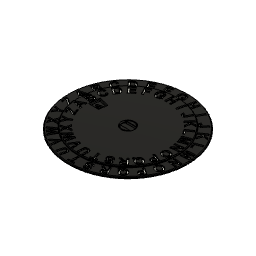
Decoder 2.0 v3 (Autodesk Fusion 360 design; units mm, degrees)
Autodesk Fusion 360 part; units mm, degrees
sketch "Sketch1" plane through (0, 0, 0) normal (0, 0, 1) x (1, 0, 0) in component "Decoder Base"
  line L0 (0, 0) -> (-75, 0)
  arc A0 (-72.8206, 17.9487) -> (-75, 0) centre (0, 0) ccw
  line L1 (0, 0) -> (-72.8206, 17.9487) construction
  line L2 (0, 0) -> (-75, 0) construction
  line L3 (-75, 0) -> (-62.5, 0)
  line L4 (-62.5, 0) -> (-50, 0)
  line L5 (-62.5, 0) -> (-61.5, 0)
  line L6 (-50, 0) -> (-37.5, 0)
  arc A1 (-60.6839, 14.9572) -> (-62.5, 0) centre (0, 0) ccw
  line L7 (0, 0) -> (-60.6839, 14.9572) construction
  line L8 (0, 0) -> (-62.5, 0) construction
  arc A2 (-48.5471, 11.9658) -> (-50, 0) centre (0, 0) ccw
  line L9 (0, 0) -> (-48.5471, 11.9658) construction
  line L10 (0, 0) -> (-50, 0) construction
  arc A3 (-36.4103, 8.9743) -> (-37.5, 0) centre (0, 0) ccw
  line L11 (0, 0) -> (-36.4103, 8.9743) construction
  line L12 (0, 0) -> (-37.5, 0) construction
  arc A4 (-59.7129, 14.7179) -> (-61.5, 0) centre (0, 0) ccw
  line L13 (0, 0) -> (-59.7129, 14.7179) construction
  line L14 (0, 0) -> (-61.5, 0) construction
  arc A5 (-61.5, 0) -> (-59.7129, -14.7179) centre (0, 0) ccw
  arc A6 (-50, 0) -> (-48.5471, -11.9658) centre (0, 0) ccw
  arc A7 (-37.5, 0) -> (-36.4103, -8.9743) centre (0, 0) ccw
  arc A8 (-62.5, 0) -> (-60.6839, -14.9572) centre (0, 0) ccw
  line L15 (-72.8206, -17.9487) -> (-60.6839, -14.9572)
  line L16 (-60.6839, -14.9572) -> (-59.7129, -14.7179)
  line L17 (-48.5471, -11.9658) -> (-36.4103, -8.9743)
  line L18 (-60.6839, -14.9572) -> (-48.5471, -11.9658)
  arc A9 (-75, 0) -> (-72.8206, -17.9487) centre (0, 0) ccw
  arc A10 (-59.7129, -14.7179) -> (-54.4555, -28.5805) centre (0, 0) ccw
  arc A11 (-48.5471, -11.9658) -> (-44.2728, -23.2362) centre (0, 0) ccw
  arc A12 (-36.4103, -8.9743) -> (-33.2046, -17.4271) centre (0, 0) ccw
  arc A13 (-60.6839, -14.9572) -> (-55.341, -29.0452) centre (0, 0) ccw
  line L19 (-66.4092, -34.8542) -> (-55.341, -29.0452)
  line L20 (-55.341, -29.0452) -> (-54.4555, -28.5805)
  line L21 (-44.2728, -23.2362) -> (-33.2046, -17.4271)
  line L22 (-55.341, -29.0452) -> (-44.2728, -23.2362)
  arc A14 (-72.8206, -17.9487) -> (-66.4092, -34.8542) centre (0, 0) ccw
  arc A15 (-54.4555, -28.5805) -> (-46.0334, -40.782) centre (0, 0) ccw
  arc A16 (-44.2728, -23.2362) -> (-37.4255, -33.1561) centre (0, 0) ccw
  arc A17 (-33.2046, -17.4271) -> (-28.0692, -24.8671) centre (0, 0) ccw
  arc A18 (-55.341, -29.0452) -> (-46.7819, -41.4452) centre (0, 0) ccw
  line L23 (-56.1383, -49.7342) -> (-46.7819, -41.4452)
  line L24 (-46.7819, -41.4452) -> (-46.0334, -40.782)
  line L25 (-37.4255, -33.1561) -> (-28.0692, -24.8671)
  line L26 (-46.7819, -41.4452) -> (-37.4255, -33.1561)
  arc A19 (-66.4092, -34.8542) -> (-56.1383, -49.7342) centre (0, 0) ccw
  arc A20 (-46.0334, -40.782) -> (-34.936, -50.6135) centre (0, 0) ccw
  arc A21 (-37.4255, -33.1561) -> (-28.4032, -41.1492) centre (0, 0) ccw
  arc A22 (-28.0692, -24.8671) -> (-21.3024, -30.8619) centre (0, 0) ccw
  arc A23 (-46.7819, -41.4452) -> (-35.504, -51.4365) centre (0, 0) ccw
  line L27 (-42.6049, -61.7238) -> (-35.504, -51.4365)
  line L28 (-35.504, -51.4365) -> (-34.936, -50.6135)
  line L29 (-28.4032, -41.1492) -> (-21.3024, -30.8619)
  line L30 (-35.504, -51.4365) -> (-28.4032, -41.1492)
  arc A24 (-56.1383, -49.7342) -> (-42.6049, -61.7238) centre (0, 0) ccw
  arc A25 (-34.936, -50.6135) -> (-21.8082, -57.5035) centre (0, 0) ccw
  arc A26 (-28.4032, -41.1492) -> (-17.7302, -46.7508) centre (0, 0) ccw
  arc A27 (-21.3024, -30.8619) -> (-13.2977, -35.0631) centre (0, 0) ccw
  arc A28 (-35.504, -51.4365) -> (-22.1628, -58.4385) centre (0, 0) ccw
  line L31 (-26.5954, -70.1262) -> (-22.1628, -58.4385)
  line L32 (-22.1628, -58.4385) -> (-21.8082, -57.5035)
  line L33 (-17.7302, -46.7508) -> (-13.2977, -35.0631)
  line L34 (-22.1628, -58.4385) -> (-17.7302, -46.7508)
  arc A29 (-42.6049, -61.7238) -> (-26.5954, -70.1262) centre (0, 0) ccw
  arc A30 (-21.8082, -57.5035) -> (-7.413, -61.0516) centre (0, 0) ccw
  arc A31 (-17.7302, -46.7508) -> (-6.0268, -49.6354) centre (0, 0) ccw
  arc A32 (-13.2977, -35.0631) -> (-4.5201, -37.2266) centre (0, 0) ccw
  arc A33 (-22.1628, -58.4385) -> (-7.5335, -62.0443) centre (0, 0) ccw
  line L35 (-9.0403, -74.4532) -> (-7.5335, -62.0443)
  line L36 (-7.5335, -62.0443) -> (-7.413, -61.0516)
  line L37 (-6.0268, -49.6354) -> (-4.5201, -37.2266)
  line L38 (-7.5335, -62.0443) -> (-6.0268, -49.6354)
  arc A34 (-26.5954, -70.1262) -> (-9.0403, -74.4532) centre (0, 0) ccw
  arc A35 (-7.413, -61.0516) -> (7.413, -61.0516) centre (0, 0) ccw
  arc A36 (-6.0268, -49.6354) -> (6.0268, -49.6354) centre (0, 0) ccw
  arc A37 (-4.5201, -37.2266) -> (4.5201, -37.2266) centre (0, 0) ccw
  arc A38 (-7.5335, -62.0443) -> (7.5335, -62.0443) centre (0, 0) ccw
  line L39 (9.0403, -74.4532) -> (7.5335, -62.0443)
  line L40 (7.5335, -62.0443) -> (7.413, -61.0516)
  line L41 (6.0268, -49.6354) -> (4.5201, -37.2266)
  line L42 (7.5335, -62.0443) -> (6.0268, -49.6354)
  arc A39 (-9.0403, -74.4532) -> (9.0403, -74.4532) centre (0, 0) ccw
  arc A40 (7.413, -61.0516) -> (21.8082, -57.5035) centre (0, 0) ccw
  arc A41 (6.0268, -49.6354) -> (17.7302, -46.7508) centre (0, 0) ccw
  arc A42 (4.5201, -37.2266) -> (13.2977, -35.0631) centre (0, 0) ccw
  arc A43 (7.5335, -62.0443) -> (22.1628, -58.4385) centre (0, 0) ccw
  line L43 (26.5954, -70.1262) -> (22.1628, -58.4385)
  line L44 (22.1628, -58.4385) -> (21.8082, -57.5035)
  line L45 (17.7302, -46.7508) -> (13.2977, -35.0631)
  line L46 (22.1628, -58.4385) -> (17.7302, -46.7508)
  arc A44 (9.0403, -74.4532) -> (26.5954, -70.1262) centre (0, 0) ccw
  arc A45 (21.8082, -57.5035) -> (34.936, -50.6135) centre (0, 0) ccw
  arc A46 (17.7302, -46.7508) -> (28.4032, -41.1492) centre (0, 0) ccw
  arc A47 (13.2977, -35.0631) -> (21.3024, -30.8619) centre (0, 0) ccw
  arc A48 (22.1628, -58.4385) -> (35.504, -51.4365) centre (0, 0) ccw
  line L47 (42.6049, -61.7238) -> (35.504, -51.4365)
  line L48 (35.504, -51.4365) -> (34.936, -50.6135)
  line L49 (28.4032, -41.1492) -> (21.3024, -30.8619)
  line L50 (35.504, -51.4365) -> (28.4032, -41.1492)
  arc A49 (26.5954, -70.1262) -> (42.6049, -61.7238) centre (0, 0) ccw
  arc A50 (34.936, -50.6135) -> (46.0334, -40.782) centre (0, 0) ccw
  arc A51 (28.4032, -41.1492) -> (37.4255, -33.1561) centre (0, 0) ccw
  arc A52 (21.3024, -30.8619) -> (28.0692, -24.8671) centre (0, 0) ccw
  arc A53 (35.504, -51.4365) -> (46.7819, -41.4452) centre (0, 0) ccw
  line L51 (56.1383, -49.7342) -> (46.7819, -41.4452)
  line L52 (46.7819, -41.4452) -> (46.0334, -40.782)
  line L53 (37.4255, -33.1561) -> (28.0692, -24.8671)
  line L54 (46.7819, -41.4452) -> (37.4255, -33.1561)
  arc A54 (42.6049, -61.7238) -> (56.1383, -49.7342) centre (0, 0) ccw
  arc A55 (46.0334, -40.782) -> (54.4555, -28.5805) centre (0, 0) ccw
  arc A56 (37.4255, -33.1561) -> (44.2728, -23.2362) centre (0, 0) ccw
  arc A57 (28.0692, -24.8671) -> (33.2046, -17.4271) centre (0, 0) ccw
  arc A58 (46.7819, -41.4452) -> (55.341, -29.0452) centre (0, 0) ccw
  line L55 (66.4092, -34.8542) -> (55.341, -29.0452)
  line L56 (55.341, -29.0452) -> (54.4555, -28.5805)
  line L57 (44.2728, -23.2362) -> (33.2046, -17.4271)
  line L58 (55.341, -29.0452) -> (44.2728, -23.2362)
  arc A59 (56.1383, -49.7342) -> (66.4092, -34.8542) centre (0, 0) ccw
  arc A60 (54.4555, -28.5805) -> (59.7129, -14.7179) centre (0, 0) ccw
  arc A61 (44.2728, -23.2362) -> (48.5471, -11.9658) centre (0, 0) ccw
  arc A62 (33.2046, -17.4271) -> (36.4103, -8.9743) centre (0, 0) ccw
  arc A63 (55.341, -29.0452) -> (60.6839, -14.9572) centre (0, 0) ccw
  line L59 (72.8206, -17.9487) -> (60.6839, -14.9572)
  line L60 (60.6839, -14.9572) -> (59.7129, -14.7179)
  line L61 (48.5471, -11.9658) -> (36.4103, -8.9743)
  line L62 (60.6839, -14.9572) -> (48.5471, -11.9658)
  arc A64 (66.4092, -34.8542) -> (72.8206, -17.9487) centre (0, 0) ccw
  arc A65 (59.7129, -14.7179) -> (61.5, 0) centre (0, 0) ccw
  arc A66 (48.5471, -11.9658) -> (50, 0) centre (0, 0) ccw
  arc A67 (36.4103, -8.9743) -> (37.5, 0) centre (0, 0) ccw
  arc A68 (60.6839, -14.9572) -> (62.5, 0) centre (0, 0) ccw
  line L63 (75, 0) -> (62.5, 0)
  line L64 (62.5, 0) -> (61.5, 0)
  line L65 (50, 0) -> (37.5, 0)
  line L66 (62.5, 0) -> (50, 0)
  arc A69 (72.8206, -17.9487) -> (75, 0) centre (0, 0) ccw
  arc A70 (61.5, 0) -> (59.7129, 14.7179) centre (0, 0) ccw
  arc A71 (50, 0) -> (48.5471, 11.9658) centre (0, 0) ccw
  arc A72 (37.5, 0) -> (36.4103, 8.9743) centre (0, 0) ccw
  arc A73 (62.5, 0) -> (60.6839, 14.9572) centre (0, 0) ccw
  line L67 (72.8206, 17.9487) -> (60.6839, 14.9572)
  line L68 (60.6839, 14.9572) -> (59.7129, 14.7179)
  line L69 (48.5471, 11.9658) -> (36.4103, 8.9743)
  line L70 (60.6839, 14.9572) -> (48.5471, 11.9658)
  arc A74 (75, 0) -> (72.8206, 17.9487) centre (0, 0) ccw
  arc A75 (59.7129, 14.7179) -> (54.4555, 28.5805) centre (0, 0) ccw
  arc A76 (48.5471, 11.9658) -> (44.2728, 23.2362) centre (0, 0) ccw
  arc A77 (36.4103, 8.9743) -> (33.2046, 17.4271) centre (0, 0) ccw
  arc A78 (60.6839, 14.9572) -> (55.341, 29.0452) centre (0, 0) ccw
  line L71 (66.4092, 34.8542) -> (55.341, 29.0452)
  line L72 (55.341, 29.0452) -> (54.4555, 28.5805)
  line L73 (44.2728, 23.2362) -> (33.2046, 17.4271)
  line L74 (55.341, 29.0452) -> (44.2728, 23.2362)
  arc A79 (72.8206, 17.9487) -> (66.4092, 34.8542) centre (0, 0) ccw
  arc A80 (54.4555, 28.5805) -> (46.0334, 40.782) centre (0, 0) ccw
  arc A81 (44.2728, 23.2362) -> (37.4255, 33.1561) centre (0, 0) ccw
  arc A82 (33.2046, 17.4271) -> (28.0692, 24.8671) centre (0, 0) ccw
  arc A83 (55.341, 29.0452) -> (46.7819, 41.4452) centre (0, 0) ccw
  line L75 (56.1383, 49.7342) -> (46.7819, 41.4452)
  line L76 (46.7819, 41.4452) -> (46.0334, 40.782)
  line L77 (37.4255, 33.1561) -> (28.0692, 24.8671)
  line L78 (46.7819, 41.4452) -> (37.4255, 33.1561)
  arc A84 (66.4092, 34.8542) -> (56.1383, 49.7342) centre (0, 0) ccw
  arc A85 (46.0334, 40.782) -> (34.936, 50.6135) centre (0, 0) ccw
  arc A86 (37.4255, 33.1561) -> (28.4032, 41.1492) centre (0, 0) ccw
  arc A87 (28.0692, 24.8671) -> (21.3024, 30.8619) centre (0, 0) ccw
  arc A88 (46.7819, 41.4452) -> (35.504, 51.4365) centre (0, 0) ccw
  line L79 (42.6049, 61.7238) -> (35.504, 51.4365)
  line L80 (35.504, 51.4365) -> (34.936, 50.6135)
  line L81 (28.4032, 41.1492) -> (21.3024, 30.8619)
  line L82 (35.504, 51.4365) -> (28.4032, 41.1492)
  arc A89 (56.1383, 49.7342) -> (42.6049, 61.7238) centre (0, 0) ccw
  arc A90 (34.936, 50.6135) -> (21.8082, 57.5035) centre (0, 0) ccw
  arc A91 (28.4032, 41.1492) -> (17.7302, 46.7508) centre (0, 0) ccw
  arc A92 (21.3024, 30.8619) -> (13.2977, 35.0631) centre (0, 0) ccw
  arc A93 (35.504, 51.4365) -> (22.1628, 58.4385) centre (0, 0) ccw
  line L83 (26.5954, 70.1262) -> (22.1628, 58.4385)
  line L84 (22.1628, 58.4385) -> (21.8082, 57.5035)
  line L85 (17.7302, 46.7508) -> (13.2977, 35.0631)
  line L86 (22.1628, 58.4385) -> (17.7302, 46.7508)
  arc A94 (42.6049, 61.7238) -> (26.5954, 70.1262) centre (0, 0) ccw
  arc A95 (21.8082, 57.5035) -> (7.413, 61.0516) centre (0, 0) ccw
  arc A96 (17.7302, 46.7508) -> (6.0268, 49.6354) centre (0, 0) ccw
  arc A97 (13.2977, 35.0631) -> (4.5201, 37.2266) centre (0, 0) ccw
  arc A98 (22.1628, 58.4385) -> (7.5335, 62.0443) centre (0, 0) ccw
  line L87 (9.0403, 74.4532) -> (7.5335, 62.0443)
  line L88 (7.5335, 62.0443) -> (7.413, 61.0516)
  line L89 (6.0268, 49.6354) -> (4.5201, 37.2266)
  line L90 (7.5335, 62.0443) -> (6.0268, 49.6354)
  arc A99 (26.5954, 70.1262) -> (9.0403, 74.4532) centre (0, 0) ccw
  arc A100 (7.413, 61.0516) -> (-7.413, 61.0516) centre (0, 0) ccw
  arc A101 (6.0268, 49.6354) -> (-6.0268, 49.6354) centre (0, 0) ccw
  arc A102 (4.5201, 37.2266) -> (-4.5201, 37.2266) centre (0, 0) ccw
  arc A103 (7.5335, 62.0443) -> (-7.5335, 62.0443) centre (0, 0) ccw
  line L91 (-9.0403, 74.4532) -> (-7.5335, 62.0443)
  line L92 (-7.5335, 62.0443) -> (-7.413, 61.0516)
  line L93 (-6.0268, 49.6354) -> (-4.5201, 37.2266)
  line L94 (-7.5335, 62.0443) -> (-6.0268, 49.6354)
  arc A104 (9.0403, 74.4532) -> (-9.0403, 74.4532) centre (0, 0) ccw
  arc A105 (-7.413, 61.0516) -> (-21.8082, 57.5035) centre (0, 0) ccw
  arc A106 (-6.0268, 49.6354) -> (-17.7302, 46.7508) centre (0, 0) ccw
  arc A107 (-4.5201, 37.2266) -> (-13.2977, 35.0631) centre (0, 0) ccw
  arc A108 (-7.5335, 62.0443) -> (-22.1628, 58.4385) centre (0, 0) ccw
  line L95 (-26.5954, 70.1262) -> (-22.1628, 58.4385)
  line L96 (-22.1628, 58.4385) -> (-21.8082, 57.5035)
  line L97 (-17.7302, 46.7508) -> (-13.2977, 35.0631)
  line L98 (-22.1628, 58.4385) -> (-17.7302, 46.7508)
  arc A109 (-9.0403, 74.4532) -> (-26.5954, 70.1262) centre (0, 0) ccw
  arc A110 (-21.8082, 57.5035) -> (-34.936, 50.6135) centre (0, 0) ccw
  arc A111 (-17.7302, 46.7508) -> (-28.4032, 41.1492) centre (0, 0) ccw
  arc A112 (-13.2977, 35.0631) -> (-21.3024, 30.8619) centre (0, 0) ccw
  arc A113 (-22.1628, 58.4385) -> (-35.504, 51.4365) centre (0, 0) ccw
  line L99 (-42.6049, 61.7238) -> (-35.504, 51.4365)
  line L100 (-35.504, 51.4365) -> (-34.936, 50.6135)
  line L101 (-28.4032, 41.1492) -> (-21.3024, 30.8619)
  line L102 (-35.504, 51.4365) -> (-28.4032, 41.1492)
  arc A114 (-26.5954, 70.1262) -> (-42.6049, 61.7238) centre (0, 0) ccw
  arc A115 (-34.936, 50.6135) -> (-46.0334, 40.782) centre (0, 0) ccw
  arc A116 (-28.4032, 41.1492) -> (-37.4255, 33.1561) centre (0, 0) ccw
  arc A117 (-21.3024, 30.8619) -> (-28.0692, 24.8671) centre (0, 0) ccw
  arc A118 (-35.504, 51.4365) -> (-46.7819, 41.4452) centre (0, 0) ccw
  line L103 (-56.1383, 49.7342) -> (-46.7819, 41.4452)
  line L104 (-46.7819, 41.4452) -> (-46.0334, 40.782)
  line L105 (-37.4255, 33.1561) -> (-28.0692, 24.8671)
  line L106 (-46.7819, 41.4452) -> (-37.4255, 33.1561)
  arc A119 (-42.6049, 61.7238) -> (-56.1383, 49.7342) centre (0, 0) ccw
  arc A120 (-46.0334, 40.782) -> (-54.4555, 28.5805) centre (0, 0) ccw
  arc A121 (-37.4255, 33.1561) -> (-44.2728, 23.2362) centre (0, 0) ccw
  arc A122 (-28.0692, 24.8671) -> (-33.2046, 17.4271) centre (0, 0) ccw
  arc A123 (-46.7819, 41.4452) -> (-55.341, 29.0452) centre (0, 0) ccw
  line L107 (-66.4092, 34.8542) -> (-55.341, 29.0452)
  line L108 (-55.341, 29.0452) -> (-54.4555, 28.5805)
  line L109 (-44.2728, 23.2362) -> (-33.2046, 17.4271)
  line L110 (-55.341, 29.0452) -> (-44.2728, 23.2362)
  arc A124 (-56.1383, 49.7342) -> (-66.4092, 34.8542) centre (0, 0) ccw
  arc A125 (-54.4555, 28.5805) -> (-59.7129, 14.7179) centre (0, 0) ccw
  arc A126 (-44.2728, 23.2362) -> (-48.5471, 11.9658) centre (0, 0) ccw
  arc A127 (-33.2046, 17.4271) -> (-36.4103, 8.9743) centre (0, 0) ccw
  arc A128 (-55.341, 29.0452) -> (-60.6839, 14.9572) centre (0, 0) ccw
  line L111 (-72.8206, 17.9487) -> (-60.6839, 14.9572)
  line L112 (-60.6839, 14.9572) -> (-59.7129, 14.7179)
  line L113 (-48.5471, 11.9658) -> (-36.4103, 8.9743)
  line L114 (-60.6839, 14.9572) -> (-48.5471, 11.9658)
  arc A129 (-66.4092, 34.8542) -> (-72.8206, 17.9487) centre (0, 0) ccw
  line L115 (-37.5, 0) -> (-36.5, 0)
  arc A130 (-35.4394, 8.735) -> (-36.5, 0) centre (0, 0) ccw
  line L116 (0, 0) -> (-35.4394, 8.735) construction
  line L117 (0, 0) -> (-36.5, 0) construction
  line L118 (-36.4103, 8.9743) -> (-35.4394, 8.735)
  line L119 (-50, 0) -> (-48, 0)
  line L120 (-48.5471, 11.9658) -> (-46.6052, 11.4872)
  arc A131 (-46.6052, 11.4872) -> (-48, 0) centre (0, 0) ccw
  circle A132 centre (0, 0) radius 7.5
  circle A133 centre (0, 0) radius 17.5
  dimension "d1" = 75
  dimension "d2" = 13.846
  dimension "d5" = 12.5
  dimension "d6" = 12.5
  dimension "d7" = 1
  dimension "d8" = 12.5
  dimension "d9" = 13.846
  dimension "d10" = 13.846
  dimension "d11" = 10
  dimension "d12" = 10
  dimension "d13" = 13.846
  dimension "d14" = 8.5
  dimension "d15" = 13.846
  dimension "d17" = 360
  dimension "d18" = 10
  dimension "d19" = 10
  dimension "d20" = 10
  dimension "d21" = 10
  dimension "d22" = 10
  dimension "d23" = 10
  dimension "d24" = 10
  dimension "d25" = 10
  dimension "d26" = 10
  dimension "d27" = 10
  dimension "d28" = 10
  dimension "d29" = 10
  dimension "d30" = 10
  dimension "d31" = 10
  dimension "d32" = 10
  dimension "d33" = 10
  dimension "d34" = 10
  dimension "d35" = 10
  dimension "d36" = 10
  dimension "d37" = 10
  dimension "d38" = 10
  dimension "d39" = 10
  dimension "d40" = 10
  dimension "d41" = 10
  dimension "d42" = 10
  dimension "d43" = 10
  dimension "d44" = 10
  dimension "d45" = 10
  dimension "d46" = 10
  dimension "d47" = 10
  dimension "d48" = 10
  dimension "d49" = 10
  dimension "d50" = 10
  dimension "d51" = 10
  dimension "d52" = 10
  dimension "d53" = 10
  dimension "d54" = 10
  dimension "d55" = 10
  dimension "d56" = 10
  dimension "d57" = 8.5
  dimension "d58" = 8.5
  dimension "d59" = 8.5
  dimension "d60" = 8.5
  dimension "d61" = 8.5
  dimension "d62" = 8.5
  dimension "d63" = 8.5
  dimension "d64" = 8.5
  dimension "d65" = 8.5
  dimension "d66" = 8.5
  dimension "d67" = 8.5
  dimension "d68" = 8.5
  dimension "d69" = 8.5
  dimension "d70" = 8.5
  dimension "d71" = 8.5
  dimension "d72" = 8.5
  dimension "d73" = 8.5
  dimension "d74" = 8.5
  dimension "d75" = 8.5
  dimension "d76" = 8.5
  dimension "d77" = 8.5
  dimension "d78" = 8.5
  dimension "d79" = 8.5
  dimension "d80" = 8.5
  dimension "d81" = 8.5
  dimension "d82" = 10
  dimension "d83" = 10
  dimension "d84" = 10
  dimension "d85" = 10
  dimension "d86" = 10
  dimension "d87" = 10
  dimension "d88" = 10
  dimension "d89" = 10
  dimension "d90" = 10
  dimension "d91" = 10
  dimension "d92" = 10
  dimension "d93" = 1
  dimension "d94" = 13.846
  dimension "d95" = 2
  dimension "d96" = 2
  dimension "d97" = 15
  dimension "d98" = 35
  text T0 "A" font "Arial" height 10 bold align centre spacing 1 along the path A1 letters at x, y, angle (-75.2068, 4.0504, 83.0769)
  text T1 "B" font "Arial" height 10 bold align centre spacing 1 along the path A2 letters at x, y, angle (-62.7979, 2.5437, 83.0769)
  text T2 "A" font "Arial" height 8.5 bold align centre spacing 1 along the path A3 letters at x, y, angle (-48.4147, 1.5594, 83.0769)
  text T3 "B" font "Arial" height 10 bold align centre spacing 1 along the path A128 letters at x, y, angle (-72.0521, 21.9308, 69.2308)
  text T4 "C" font "Arial" height 10 bold align centre spacing 1 along the path A126 letters at x, y, angle (-60.3644, 17.4983, 69.2308)
  text T5 "D" font "Arial" height 10 bold align centre spacing 1 along the path A121 letters at x, y, angle (-54.4227, 31.4359, 55.3846)
  text T6 "E" font "Arial" height 10 bold align centre spacing 1 along the path A116 letters at x, y, angle (-45.0297, 43.8023, 41.5385)
  text T7 "F" font "Arial" height 10 bold align centre spacing 1 along the path A111 letters at x, y, angle (-32.8913, 53.488, 27.6923)
  text T8 "G" font "Arial" height 10 bold align centre spacing 1 along the path A106 letters at x, y, angle (-20.2676, 59.526, 13.8462)
  text T9 "H" font "Arial" height 10 bold align centre spacing 1 along the path A101 letters at x, y, angle (-5.0443, 62.6467, 0)
  text T10 "I" font "Arial" height 10 bold align centre spacing 1 along the path A96 letters at x, y, angle (13.1081, 61.2907, -13.8462)
  text T11 "J" font "Arial" height 10 bold align centre spacing 1 along the path A91 letters at x, y, angle (25.6736, 57.2762, -27.6923)
  text T12 "K" font "Arial" height 10 bold align centre spacing 1 along the path A86 letters at x, y, angle (37.7667, 50.2367, -41.5385)
  text T13 "L" font "Arial" height 10 bold align centre spacing 1 along the path A81 letters at x, y, angle (49.1334, 39.0988, -55.3846)
  text T14 "M" font "Arial" height 10 bold align centre spacing 1 along the path A76 letters at x, y, angle (56.5124, 27.6553, -69.2308)
  text T15 "N" font "Arial" height 10 bold align centre spacing 1 along the path A71 letters at x, y, angle (61.5819, 12.5588, -83.0769)
  text T16 "O" font "Arial" height 10 bold align centre spacing 1 along the path A66 letters at x, y, angle (62.8448, -2.1577, -96.9231)
  text T17 "P" font "Arial" height 10 bold align centre spacing 1 along the path A61 letters at x, y, angle (60.2277, -17.8586, -110.7692)
  text T18 "Q" font "Arial" height 10 bold align centre spacing 1 along the path A56 letters at x, y, angle (54.6436, -31.116, -124.6154)
  text T19 "R" font "Arial" height 10 bold align centre spacing 1 along the path A51 letters at x, y, angle (45.3182, -43.5467, -138.4615)
  text T20 "S" font "Arial" height 10 bold align centre spacing 1 along the path A46 letters at x, y, angle (33.2386, -53.3057, -152.3077)
  text T21 "T" font "Arial" height 10 bold align centre spacing 1 along the path A41 letters at x, y, angle (19.1351, -59.8052, -166.1538)
  text T22 "U" font "Arial" height 10 bold align centre spacing 1 along the path A36 letters at x, y, angle (5.0443, -62.6467, 180)
  text T23 "V" font "Arial" height 10 bold align centre spacing 1 along the path A31 letters at x, y, angle (-10.4655, -61.942, 166.1538)
  text T24 "W" font "Arial" height 10 bold align centre spacing 1 along the path A26 letters at x, y, angle (-23.2757, -58.5347, 152.3077)
  text T25 "X" font "Arial" height 10 bold align centre spacing 1 along the path A21 letters at x, y, angle (-38.0552, -49.9811, 138.4615)
  text T26 "Y" font "Arial" height 10 bold align centre spacing 1 along the path A16 letters at x, y, angle (-48.9009, -39.4356, 124.6154)
  text T27 "Z" font "Arial" height 10 bold align centre spacing 1 along the path A11 letters at x, y, angle (-57.0626, -26.2043, 110.7692)
  text T28 "A" font "Arial" height 10 bold align centre spacing 1 along the path A6 letters at x, y, angle (-61.5819, -12.5588, 96.9231)
  text T29 "Z" font "Arial" height 10 bold align centre spacing 1 along the path A8 letters at x, y, angle (-74.0845, -13.2935, 96.9231)
  text T30 "Y" font "Arial" height 10 bold align centre spacing 1 along the path A13 letters at x, y, angle (-68.6052, -31.0195, 110.7692)
  text T31 "X" font "Arial" height 10 bold align centre spacing 1 along the path A18 letters at x, y, angle (-59.1979, -46.5224, 124.6154)
  text T32 "W" font "Arial" height 10 bold align centre spacing 1 along the path A23 letters at x, y, angle (-44.8967, -60.6199, 138.4615)
  text T33 "V" font "Arial" height 10 bold align centre spacing 1 along the path A28 letters at x, y, angle (-30.7941, -68.7058, 152.3077)
  text T34 "U" font "Arial" height 10 bold align centre spacing 1 along the path A33 letters at x, y, angle (-13.086, -74.1702, 166.1538)
  text T35 "T" font "Arial" height 10 bold align centre spacing 1 along the path A38 letters at x, y, angle (4.2667, -75.1467, 180)
  text T36 "S" font "Arial" height 10 bold align centre spacing 1 along the path A43 letters at x, y, angle (22.5073, -71.8481, -166.1538)
  text T37 "R" font "Arial" height 10 bold align centre spacing 1 along the path A48 letters at x, y, angle (39.3889, -64.1948, -152.3077)
  text T38 "Q" font "Arial" height 10 bold align centre spacing 1 along the path A53 letters at x, y, angle (53.8982, -52.6452, -138.4615)
  text T39 "P" font "Arial" height 10 bold align centre spacing 1 along the path A58 letters at x, y, angle (64.4911, -38.8539, -124.6154)
  text T40 "O" font "Arial" height 10 bold align centre spacing 1 along the path A63 letters at x, y, angle (72.19, -21.5673, -110.7692)
  text T41 "N" font "Arial" height 10 bold align centre spacing 1 along the path A68 letters at x, y, angle (75.2068, -4.0504, -96.9231)
  text T42 "B" font "Arial" height 8.5 bold align centre spacing 1 along the path A7 letters at x, y, angle (-47.381, -10.0723, 96.9231)
  text T43 "C" font "Arial" height 8.5 bold align centre spacing 1 along the path A12 letters at x, y, angle (-43.5938, -21.1186, 110.7692)
  text T44 "D" font "Arial" height 8.5 bold align centre spacing 1 along the path A17 letters at x, y, angle (-37.273, -30.9376, 124.6154)
  text T45 "E" font "Arial" height 8.5 bold align centre spacing 1 along the path A22 letters at x, y, angle (-29.0313, -38.7414, 138.4615)
  text T46 "F" font "Arial" height 8.5 bold align centre spacing 1 along the path A27 letters at x, y, angle (-19.2114, -44.4084, 152.3077)
  text T47 "G" font "Arial" height 8.5 bold align centre spacing 1 along the path A32 letters at x, y, angle (-7.0629, -47.9528, 166.1538)
  text T48 "H" font "Arial" height 8.5 bold align centre spacing 1 along the path A37 letters at x, y, angle (4.2877, -48.2497, -180)
  text T49 "I" font "Arial" height 8.5 bold align centre spacing 1 along the path A42 letters at x, y, angle (13.1485, -46.4528, -166.1538)
  text T50 "J" font "Arial" height 8.5 bold align centre spacing 1 along the path A47 letters at x, y, angle (25.3465, -41.1884, -152.3077)
  text T51 "K" font "Arial" height 8.5 bold align centre spacing 1 along the path A52 letters at x, y, angle (35.2048, -33.2721, -138.4615)
  text T52 "L" font "Arial" height 8.5 bold align centre spacing 1 along the path A57 letters at x, y, angle (41.7689, -24.4242, -124.6154)
  text T53 "M" font "Arial" height 8.5 bold align centre spacing 1 along the path A62 letters at x, y, angle (46.868, -12.4852, -110.7692)
  text T54 "N" font "Arial" height 8.5 bold align centre spacing 1 along the path A67 letters at x, y, angle (48.4147, -1.5594, -96.9231)
  text T55 "Z" font "Arial" height 8.5 bold align centre spacing 1 along the path A127 letters at x, y, angle (-46.4003, 13.7185, 69.2308)
  text T56 "O" font "Arial" height 8.5 bold align centre spacing 1 along the path A72 letters at x, y, angle (47.3412, 10.4004, -83.0769)
  text T57 "P" font "Arial" height 8.5 bold align centre spacing 1 along the path A77 letters at x, y, angle (43.7099, 20.8123, -69.2308)
  text T58 "Q" font "Arial" height 8.5 bold align centre spacing 1 along the path A82 letters at x, y, angle (37.0853, 31.2096, -55.3846)
  text T59 "R" font "Arial" height 8.5 bold align centre spacing 1 along the path A87 letters at x, y, angle (28.7861, 38.9587, -41.5385)
  text T60 "S" font "Arial" height 8.5 bold align centre spacing 1 along the path A92 letters at x, y, angle (18.9162, 44.5633, -27.6923)
  text T61 "T" font "Arial" height 8.5 bold align centre spacing 1 along the path A97 letters at x, y, angle (8.0256, 47.7155, -13.8462)
  text T62 "U" font "Arial" height 8.5 bold align centre spacing 1 along the path A102 letters at x, y, angle (-4.2877, 48.2497, 0)
  text T63 "V" font "Arial" height 8.5 bold align centre spacing 1 along the path A107 letters at x, y, angle (-15.3947, 45.8992, 13.8462)
  text T64 "W" font "Arial" height 8.5 bold align centre spacing 1 along the path A112 letters at x, y, angle (-27.3847, 40.1187, 27.6923)
  text T65 "X" font "Arial" height 8.5 bold align centre spacing 1 along the path A117 letters at x, y, angle (-34.9596, 33.4894, 41.5385)
  text T66 "Y" font "Arial" height 8.5 bold align centre spacing 1 along the path A122 letters at x, y, angle (-41.9665, 24.1379, 55.3846)
  text T67 "C" font "Arial" height 10 bold align centre spacing 1 along the path A123 letters at x, y, angle (-64.71, 38.5368, 55.3846)
  text T68 "D" font "Arial" height 10 bold align centre spacing 1 along the path A118 letters at x, y, angle (-53.6072, 52.9031, 41.5385)
  text T69 "E" font "Arial" height 10 bold align centre spacing 1 along the path A113 letters at x, y, angle (-39.0477, 64.3739, 27.6923)
  text T70 "F" font "Arial" height 10 bold align centre spacing 1 along the path A108 letters at x, y, angle (-22.1265, 71.9419, 13.8462)
  text T71 "G" font "Arial" height 10 bold align centre spacing 1 along the path A103 letters at x, y, angle (-5.4332, 75.1467, 0)
  text T72 "H" font "Arial" height 10 bold align centre spacing 1 along the path A98 letters at x, y, angle (13.086, 74.1702, -13.8462)
  text T73 "I" font "Arial" height 10 bold align centre spacing 1 along the path A93 letters at x, y, angle (33.204, 67.4409, -27.6923)
  text T74 "J" font "Arial" height 10 bold align centre spacing 1 along the path A88 letters at x, y, angle (46.9237, 58.8241, -41.5385)
  text T75 "K" font "Arial" height 10 bold align centre spacing 1 along the path A83 letters at x, y, angle (58.979, 46.8396, -55.3846)
  text T76 "L" font "Arial" height 10 bold align centre spacing 1 along the path A78 letters at x, y, angle (68.7503, 30.6368, -69.2308)
  text T77 "M" font "Arial" height 10 bold align centre spacing 1 along the path A73 letters at x, y, angle (73.8974, 14.8341, -83.0769)
  constraint coincident L0.start A0.centre
  constraint horizontal L0
  constraint parallel L0 L3
  constraint parallel L0 L4
  constraint parallel L2 L5
  constraint parallel L0 L6
  constraint horizontal L115
  constraint parallel L10 L119
  constraint parallel L113 L120
  constraint concentric A95 A132
  constraint concentric A52 A133
  measures "d1" distance of L0.start L0.end
  measures "d2" angle of L1 L2
  measures "d5" distance of L0.end L3.end
  measures "d6" distance of L3.end L4.end
  measures "d7" distance of L3.end L5.end
  measures "d8" distance of L4.end L6.end
  measures "d9" angle of L7 L8
  measures "d10" angle of L9 L10
  measures "d13" angle of L11 L12
  measures "d15" angle of L13 L14
  measures "d93" distance of L6.end L115.end
  measures "d94" angle of L116 L117
  measures "d95" distance of L4.end L119.end
  measures "d96" distance of A2.start L120.end
  measures "d97" diameter of A132
  measures "d98" diameter of A133
extrude "Extrude1" add sketch "Sketch1" sketch "Sketch1" along normal blind 2.5 contours L0 A7 A12 A17 A22 A27 A32 A37 A42 A47 A52 A57 A62 A67 A72 A77 A82 A87 A92 A97 A102 A107 A112 A117 A122 A127 L115 A130 L118 | L0 A3 L115 A130 L118 | L0 L6 A6 A7 L17 L119 | L0 L6 A3 L113 A131 | L0 L6 A2 L113 L119 L120 A131 | L109 A126 A127 L113 L120 | L17 A11 A12 L21 | L0 L4 A5 A6 L18 | L0 L4 A2 A4 L114 | L105 A121 A122 L109 | L18 A10 A11 L22 | L21 A16 A17 L25 | L0 L4 L5 A5 A8 L16 L18 | L0 L4 L5 A1 A4 L112 L114 | L110 A125 A126 L114 | L101 A116 A117 L105 | L106 A120 A121 L110 | L16 L18 A10 A13 L20 L22 | L22 A15 A16 L26 | L25 A21 A22 L29 | L0 L3 A8 L15 A9 | L0 A0 L3 A1 L111 | L108 L110 A125 A128 L112 L114 | L97 A111 A112 L101 | L102 A115 A116 L106 | L104 L106 A120 A123 L108 L110 | L15 A13 L19 A14 | L20 L22 A15 A18 L24 L26 | L26 A20 A21 L30 | L29 A26 A27 L33 | L107 A128 L111 A129 | L93 A106 A107 L97 | L98 A110 A111 L102 | L100 L102 A115 A118 L104 L106 | L103 A123 L107 A124 | L19 A18 L23 A19 | L24 L26 A20 A23 L28 L30 | L30 A25 A26 L34 | L33 A31 A32 L37 | L89 A101 A102 L93 | L94 A105 A106 L98 | L96 L98 A110 A113 L100 L102 | L99 A118 L103 A119 | L23 A23 L27 A24 | L28 L30 A25 A28 L32 L34 | L34 A30 A31 L38 | L37 A36 A37 L41 | L85 A96 A97 L89 | L90 A100 A101 L94 | L92 L94 A105 A108 L96 L98 | L95 A113 L99 A114 | L27 A28 L31 A29 | L32 L34 A30 A33 L36 L38 | L38 A35 A36 L42 | L41 A41 A42 L45 | L81 A91 A92 L85 | L86 A95 A96 L90 | L88 L90 A100 A103 L92 L94 | L91 A108 L95 A109 | L31 A33 L35 A34 | L36 L38 A35 A38 L40 L42 | L42 A40 A41 L46 | L45 A46 A47 L49 | L77 A86 A87 L81 | L82 A90 A91 L86 | L84 L86 A95 A98 L88 L90 | L87 A103 L91 A104 | L35 A38 L39 A39 | L40 L42 A40 A43 L44 L46 | L46 A45 A46 L50 | L49 A51 A52 L53 | L73 A81 A82 L77 | L78 A85 A86 L82 | L80 L82 A90 A93 L84 L86 | L83 A98 L87 A99 | L39 A43 L43 A44 | L44 L46 A45 A48 L48 L50 | L50 A50 A51 L54 | L53 A56 A57 L57 | L69 A76 A77 L73 | L74 A80 A81 L78 | L76 L78 A85 A88 L80 L82 | L79 A93 L83 A94 | L43 A48 L47 A49 | L48 L50 A50 A53 L52 L54 | L54 A55 A56 L58 | L57 A61 A62 L61 | L65 A71 A72 L69 | L70 A75 A76 L74 | L72 L74 A80 A83 L76 L78 | L75 A88 L79 A89 | L47 A53 L51 A54 | L52 L54 A55 A58 L56 L58 | L58 A60 A61 L62 | L61 A66 A67 L65 | L66 A70 A71 L70 | L68 L70 A75 A78 L72 L74 | L71 A83 L75 A84 | L51 A58 L55 A59 | L56 L58 A60 A63 L60 L62 | L62 A65 A66 L66 | L64 L66 A70 A73 L68 L70 | L67 A78 L71 A79 | L55 A63 L59 A64 | L60 L62 A65 A68 L64 L66 | L63 A73 L67 A74 | L59 A68 L63 A69 | A132 | A133 of sketch 2 text T30 T18 T61 T48 T41 T44 T11 T40 T38 T37 T42 T39 T7 T8 T70 T46 T73 T56 T71 T57 T47 T54 T33 T59 T45 T75 T9 T3 T21 T58 T69 T2 T16 T77 T35 T1 T10 T23 T63 T65 T19 T12 T60 T62 T55 T5 T24 T26 T0 T13 T31 T14 T6 T50 T28 T49 T17 T34 T20 T15 T32 T53 T36 T27 T29 T51 T52 T43 T74 T66 T72 T25 T64 T67 T22 T68 T76 T4 makes body 1 in component "Decoder Base"
extrude "Extrude2" cut sketch "Sketch1" against normal blind 1.5 from surface at 2.5 text T0 T29 T30 T31 T32 T33 T34 T35 T36 T37 T38 T39 T40 T41 T54 T53 T52 T50 T49 T48 T47 T46 T45 T44 T43 T42 T55 T66 T65 T64 T63 T62 T61 T60 T59 T58 T57 T56 T3 T67 T68 T69 T70 T71 T72 T73 T74 T75 T76 T77 T51 T2 bodies 1 in component "Decoder Base"
sketch "Sketch2" plane through (0, 0, 0) normal (1, 0, 0) x (0, 1, 0) in component "Decoder Base"
  line L0 (0, 0) -> (7.5, 0)
  line L1 (7.5, 0) -> (7.5, 2.5)
  line L2 (7.5, 2.5) -> (7.5, 2.75)
  line L3 (7.5, 2.75) -> (7.5, 5.25)
  line L4 (7.5, 5.25) -> (8.5, 5.25)
  line L5 (7.5, 5.25) -> (7.5, 4.25)
  line L6 (7.5, 4.25) -> (8.5, 5.25)
  line L7 (7.5, 5.25) -> (8, 4.75)
  line L8 (7.5, 2.5) -> (17.5, 2.5)
  line L9 (17.5, 2.5) -> (17.5, 2.75)
  line L10 (17.5, 2.75) -> (7.5, 2.75)
  line L11 (0, 0) -> (0, 5.25)
  line L12 (0, 5.25) -> (7.5, 5.25)
  line L13 (7.5, 2.5) -> (0, 2.5)
  line L14 (7.5, 2.75) -> (0, 2.75)
  line L15 (-17.5, 2.75) -> (-7.5, 2.75)
  line L16 (-7.5, 5.25) -> (-8, 4.75)
  line L17 (-7.5, 2.5) -> (0, 2.5)
  line L18 (-7.5, 2.75) -> (0, 2.75)
  line L19 (-17.5, 2.5) -> (-17.5, 2.75)
  line L20 (0, 5.25) -> (-7.5, 5.25)
  line L21 (-7.5, 4.25) -> (-8.5, 5.25)
  line L22 (0, 0) -> (-7.5, 0)
  line L23 (-7.5, 5.25) -> (-7.5, 4.25)
  line L24 (-7.5, 5.25) -> (-8.5, 5.25)
  line L25 (-7.5, 0) -> (-7.5, 2.5)
  line L26 (-7.5, 2.5) -> (-17.5, 2.5)
  line L27 (-7.5, 2.75) -> (-7.5, 5.25)
  line L28 (-7.5, 2.5) -> (-7.5, 2.75)
  line L29 (0, 5.25) -> (3.75, 5.25)
  line L30 (0, 5.25) -> (-3.75, 5.25)
  line L31 (-3.75, 5.25) -> (-3.75, 2.5)
  line L32 (3.75, 5.25) -> (3.75, 2.5)
  dimension "d104" = 7.5
  dimension "d105" = 2.5
  dimension "d106" = 0.25
  dimension "d107" = 2.5
  dimension "d108" = 1
  dimension "d109" = 1
  dimension "d110" = 10
  dimension "d111" = 0.25
  dimension "d112" = 5.25
  constraint coincident L0.start L11.start
  constraint horizontal L0
  constraint perpendicular L0 L1
  constraint vertical L2
  constraint perpendicular L0 L3
  constraint perpendicular L3 L4
  constraint perpendicular L4 L5
  constraint midpoint L6 L7.end
  constraint perpendicular L2 L8
  constraint perpendicular L8 L9
  constraint perpendicular L0 L11
  constraint coincident L11 L13.end
  constraint perpendicular L11 L13
  constraint coincident L11 L14.end
  constraint perpendicular L11 L14
  constraint symmetric L0.start L11 L22.start
  constraint symmetric L0.end L11 L22.end
  constraint symmetric L1.end L11 L17.start
  constraint symmetric L2.end L11 L15.end
  constraint symmetric L3.end L11 L16.start
  constraint symmetric L4.end L11 L21.end
  constraint symmetric L5.end L11 L21.start
  constraint symmetric L7.end L11 L16.end
  constraint symmetric L8.end L11 L19.start
  constraint symmetric L9.end L11 L15.start
  constraint symmetric L12.start L11 L20.start
  constraint symmetric L11 L13.end L17.end
  constraint symmetric L11 L14.end L18.end
  constraint midpoint L12 L29.end
  constraint midpoint L20 L30.end
  constraint midpoint L17 L31.end
  constraint midpoint L13 L32.end
  measures "d104" distance of L0.start L0.end
  measures "d105" distance of L0.end L1.end
  measures "d106" distance of L1.end L2.end
  measures "d107" distance of L2.end L3.end
  measures "d108" distance of L3.end L4.end
  measures "d109" distance of L3.end L5.end
  measures "d110" distance of L1.end L8.end
  measures "d111" distance of L8.end L9.end
  measures "d112" distance of L0.start L11.end
sketch "Sketch3" plane through (0, 0, 0) normal (0, 0, 1) x (1, 0, 0) in component "Decoder Base"
  circle A0 centre (0, 0) radius 62
  circle A1 centre (0, 0) radius 7.5
  dimension "d113" = 124
  dimension "d114" = 15
  constraint coincident A0.centre A1.centre
  constraint concentric A0 A1
  measures "d113" diameter of A0
  measures "d114" diameter of A1
revolve "Revolve1" add sketch "Sketch2" angle 360 about axis through (0, 0, 0) along (0, 0, 1) contours L11 L13 L14 L32 | L2 L13 L14 L32 | L2 L8 L9 L10 | L11 L12 L14 L29 L32 | L3 L5 L12 L14 L32 | L3 L5 L6 L7 bodies 1 in component "Decoder Base"
extrude "Extrude3" cut sketch "Sketch2" along normal mid plane 24 contours L11 L18 L20 L30 L31 | L11 L12 L14 L29 L32 bodies 1 in component "Decoder Base"
extrude "Extrude4" add sketch "Sketch3" along normal blind 2.5 from surface at 2.75 separate body makes body 2 in component "Decoder Base"
extrude "Extrude5" cut sketch "Sketch1" against normal blind 1.5 from surface at 5.25 text T1 T4 T5 T6 T7 T8 T9 T10 T11 T12 T13 T15 T14 T16 T17 T18 T19 T20 T21 T22 T23 T24 T25 T26 T28 T27 bodies 2 in component "Decoder Base"
extrude "Extrude6" cut sketch "Sketch1" against normal blind 2.5 from surface at 5.25 contours L0 A3 L115 A130 L118 | L0 L6 A3 L113 A131 bodies 2 in component "Decoder Base"
chamfer "Chamfer1" distance 1 angle 45 2 edges at (-6.9925, 2.7121, 5.25) (-6.9925, -2.7121, 2.75) on bodies 1 2 in component "Decoder Base"
chamfer "Chamfer1" distance 0.75 angle 45 8 edges at (74.5189, -8.481, 2.5) (74.5189, -8.481, 0) (-57.8043, -22.4202, 5.25) (-47.65, 5.7858, 5.25) (-42.25, 0, 5.25) (-36.2339, 4.3996, 5.25) (-41.0223, 10.1111, 5.25) (-57.8043, 22.4202, 2.75) on bodies 1 2 in component "Decoder Base"
chamfer "Chamfer1" distance 0.25 angle 45 1 edges at (-16.3157, 6.3283, 2.75) on bodies 1 2 in component "Decoder Base"
chamfer "Chamfer1" distance 0.25 angle 45 2 edges at (0, 3.75, 5.25) (0, -3.75, 5.25) on bodies 1 2 in component "Decoder Base"
component "Decoder Base" placed x (1, 0, 0) y (0, 1, 0) z (0, 0, 1) at (0, 0, 0)
equation "d1 = OuterDiameter / 2"
equation "d2 = ( 360 / 26 ) * 1 deg"
equation "OuterDiameter = 150 mm"
equation "StepSpacing = 25 mm"
equation "d5 = StepSpacing / 2"
equation "d6 = StepSpacing / 2"
equation "d8 = StepSpacing / 2"
equation "d9 = ( 360 / 26 ) * 1 deg"
equation "d10 = ( 360 / 26 ) * 1 deg"
equation "d13 = ( 360 / 26 ) * 1 deg"
equation "d15 = ( 360 / 26 ) * 1 deg"
equation "d94 = ( 360 / 26 ) * 1 deg"
equation "d113 = OuterDiameter - StepSpacing - 1 mm"
named bodies: "Decoder Base", "Decoder Top"
